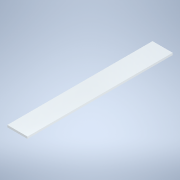
# Autodesk Inventor part: Y_Kettenhalter
Saved by Autodesk Inventor 2021 (Build 250183000, 183)
## iProperties
Created: 2021-04-26
Part Number: Y_Kettenhalter
Material: Generic
Document SubType Name: Modeling
Designer: Fabijan_Sven
Density: 1 g/cm^3
Appearance: Clear
Author: Fabijan_Sven
Autodesk Inventor part; units mm, degrees
ref_plane "YZ Plane" through (0, 0, 0) normal (1, 0, 0) x (0, 1, 0)
ref_plane "XZ Plane" through (0, 0, 0) normal (0, 1, 0) x (-1, 0, 0)
ref_plane "XY Plane" through (0, 0, 0) normal (0, 0, 1) x (1, 0, 0)
sketch "Sketch1" plane through (0, 0, 0) normal (0, 1, 0) x (-1, 0, 0)
  line L0 (0, 0) -> (63, 0)
  line L1 (63, 0) -> (63, -290)
  line L2 (63, -290) -> (0, -290)
  line L3 (0, -290) -> (0, 0)
  dimension "d0" = 290
  dimension "d1" = 63
  constraints: 8 end point, 2 parallel, 1 horizontal, 1 perpendicular
  measures "d0" distance of L0.end L1.end
  measures "d1" distance of L1.end L2.end
extrude "Extrusion1" add sketch "Sketch1" along normal blind 5
fillet "Fillet1" radius 10 2 edges at (-63, 2.5, 0) (-63, 2.5, -290)
sketch "Sketch2" plane through (0, 0, 0) normal (0, -1, 0) x (1, 0, 0)
  line L0 (-53, -251.9925) -> (-53, -308.0075) construction
  line L1 (-63, -280) -> (-63, -10) projected
  circle A0 centre (-53, -280) radius 2
  circle A1 centre (-53, -272) radius 2
  line L2 (0, -290) -> (-53, -290) projected
  point P0 (0, 0)
  dimension "d5" = 10
  dimension "d6" = 4
  dimension "d7" = 4
  dimension "d8" = 8
  dimension "d9" = 10
  constraints: 2 centre point, 2 end point, 1 midpoint, 1 point on line, 1 vertical
  measures "d5" distance between parallel lines of L0 L1
  measures "d6" diameter of A0
  measures "d7" diameter of A1
  measures "d8" distance of A1.centre A0.centre
  measures "d9" distance from line of A0.centre L2
hole "Hole1" at (-53, 0, -280) at (-53, 0, -272) direction (0, 1, 0) diameter 4 end through all
sketch "Sketch3" plane through (0, 5, 0) normal (0, 1, 0) x (1, 0, 0)
  line L0 (-10, -16.5573) -> (-10, 317.2677) construction
  line L1 (0, 0) -> (0, 290) projected
  circle A0 centre (-10, 20) radius 2.5
  circle A1 centre (-10, 270) radius 2.5
  circle A2 centre (-10, 82.5) radius 2.5
  circle A3 centre (-10, 145) radius 2.5
  line L2 (-53, 0) -> (0, 0) projected
  line L3 (0, 290) -> (-53, 290) projected
  circle A4 centre (-10, 207.5) radius 2.5
  dimension "d17" = 10
  dimension "d18" = 20
  dimension "d19" = 20
  dimension "d20" = 62.5
  dimension "d21" = 62.5
  dimension "d22" = 62.5
  dimension "d23" = 5
  dimension "d24" = 5
  dimension "d25" = 5
  dimension "d26" = 5
  dimension "d27" = 5
  constraints: 5 centre point, 5 point on line, 2 end point, 1 vertical
  measures "d17" distance between parallel lines of L1 L0
  measures "d18" distance from line of L2 A0.centre
  measures "d19" distance from line of L3 A1.centre
  measures "d20" distance of A0.centre A2.centre
  measures "d21" distance of A2.centre A3.centre
  measures "d22" distance of A3.centre A4.centre
  measures "d23" diameter of A0
  measures "d24" diameter of A2
  measures "d25" diameter of A3
  measures "d26" diameter of A4
  measures "d27" diameter of A1
hole "Hole2" at (-10, 5, -20) at (-10, 5, -82.5) at (-10, 5, -145) at (-10, 5, -207.5) at (-10, 5, -270) direction (0, -1, 0) diameter 5 end through all
equation "\"d7\" = d6"
equation "\"d10\" = d6"
equation "\"d24\" = d23"
equation "\"d25\" = d24"
equation "\"d26\" = d25"
equation "\"d27\" = d26"
equation "\"d28\" = d23"
body "Solid1"
